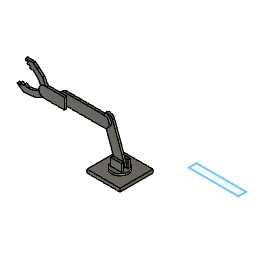
review_model_1 v2 (Autodesk Fusion 360 design; units mm, degrees)
Autodesk Fusion 360 part; units mm, degrees
note: some values were not read from the file. Set by a fixed rule: which sketch regions a step uses.
sketch "Sketch1" plane through (0, 0, 0) normal (0, 1, 0) x (1, 0, 0)
  line L0 (-108.5781, -41.3544) -> (68.499, -41.3544)
  line L1 (68.499, -41.3544) -> (68.499, 8.6456)
  line L2 (68.499, 8.6456) -> (-108.5781, 8.6456)
  line L3 (-108.5781, 8.6456) -> (-108.5781, -41.3544)
  circle A0 centre (-108.5781, -16.3544) radius 25
  circle A1 centre (68.499, -16.3544) radius 25
  circle A2 centre (-108.5781, -16.3544) radius 5
  circle A3 centre (68.499, -16.3544) radius 5
  dimension "d1" = 50
  dimension "d2" = 50
  dimension "d3" = 50
  dimension "d4" = 10
  dimension "d5" = 10
  constraint horizontal L0
  constraint vertical L1
  constraint horizontal L2
  constraint vertical L3
  constraint midpoint L3 A0.centre
  constraint midpoint L1 A1.centre
  constraint concentric A0 A2
  constraint concentric A1 A3
  measures "d1" distance of L0.start L2.end
  measures "d2" diameter of A0
  measures "d3" diameter of A1
  measures "d4" diameter of A2
  measures "d5" diameter of A3
extrude "Extrude1" add sketch "Sketch1" along normal blind 10 contours L0 L2 A0 A1 | L3 A0 A2 | L3 A0 A2 | L1 A1 A3 | L1 A1 A3 makes body 1
extrude "Extrude2" add sketch "Sketch1" along normal blind 10 and the other way blind 5 contours L3 A2 | L3 A2 bodies 1
extrude "Extrude3" add sketch "Sketch1" along normal blind 15 contours L1 A3 | L1 A3 bodies 1
sketch "Sketch2" plane through (0, 0, 0) normal (0, 0, 1) x (1, 0, 0)
  line L0 (-49.1019, 49.257) -> (100.8981, 49.257)
  line L1 (100.8981, 49.257) -> (100.8981, -100.743)
  line L2 (100.8981, -100.743) -> (-49.1019, -100.743)
  line L3 (-49.1019, -100.743) -> (-49.1019, 49.257)
  circle A0 centre (25.8981, -25.743) radius 37.5
  line L4 (44.4703, -49.3068) -> (33.9434, -49.3068)
  line L5 (33.9434, -49.3068) -> (33.9434, -0.5708)
  line L6 (33.9434, -0.5708) -> (44.4703, -0.5708)
  line L7 (44.4703, -0.5708) -> (44.4703, -49.3068)
  line L8 (14.9434, -49.3068) -> (4.8063, -49.3068)
  line L9 (4.8063, -49.3068) -> (4.8063, -0.5708)
  line L10 (4.8063, -0.5708) -> (14.9434, -0.5708)
  line L11 (14.9434, -0.5708) -> (14.9434, -49.3068)
  dimension "d14" = 150
  dimension "d15" = 150
  dimension "d19" = 75
  dimension "d24" = 19
  constraint horizontal L0
  constraint vertical L1
  constraint horizontal L2
  constraint vertical L3
  constraint horizontal L4
  constraint vertical L5
  constraint horizontal L6
  constraint vertical L7
  constraint horizontal L8
  constraint vertical L9
  constraint horizontal L10
  constraint vertical L11
  measures "d14" distance of L0.start L0.end
  measures "d15" distance of L0.start L2.end
  measures "d19" diameter of A0
  measures "d24" distance of L5 L11
copy_body "Body->Comp1" bodies 1 removing the originals makes body 2 in component "Component"
extrude "Extrude4" add sketch "Sketch2" along normal blind 15 separate body contours L0 L1 L2 L3 | A0 | L4 L5 L6 L7 | L8 L9 L10 L11 makes body 3
copy_body "Body->Comp2" bodies 3 removing the originals makes body 4 in component "Component'"
sketch "Sketch3" plane through (0, 0, 0) normal (0, 1, 0) x (1, 0, 0)
copy_body "CopyPasteBodies1" bodies 2 body 2 seen with x (1, 0, 0) y (0, 1, 0) z (0, 0, 1) at (-36.8422, -38.5395, 66.2192) makes body 5
move_body "Move1" bodies 5 to x (1, 0, 0) y (0, 1, 0) z (0, 0, 1) at (200.1869, 0, -32.8723)
copy_body "Body->Comp3" bodies 5 removing the originals makes body 6 in component "Component''"
move_body "Move1'" bodies 6 to x (0.34202, 0, -0.939693) y (0, 1, 0) z (0.939693, 0, 0.34202) at (73.7396, 0, 203.378) in component "Component''"
scale "Scale1" factor 0.881229 about (223.2311, -38.5395, 11.0656) bodies 6 in component "Component''"
extrude "Extrude1'" add sketch "Sketch2" along normal blind 10 and the other way blind -1 separate body contours A0 | L4 L5 L6 L7 | L8 L9 L10 L11 sketch seen with x (1, 0, 0) y (0, 1, 0) z (0, 0, 1) at (-0.0098, -0.0113, 15.0232) makes body 7 in component "Component'"
extrude "Extrude2'" add sketch "Sketch2" along normal blind 35 and the other way blind 5 contours L4 L5 L6 L7 | L8 L9 L10 L11 sketch seen with x (1, 0, 0) y (0, 1, 0) z (0, 0, 1) at (0.0483, -0.0113, 25.1603) bodies 7 in component "Component'"
copy_body "Body->Comp1'" bodies 7 removing the originals makes body 8 in component "Component'''"
sketch "Sketch4" plane through (0, 0, 0) normal (0, 1, 0) x (1, 0, 0)
  line L0 (94.4913, -79.8435) -> (4.0946, -79.8435)
  line L1 (4.0946, -79.8435) -> (4.0946, -29.8435)
  line L2 (4.0946, -29.8435) -> (94.4913, -29.8435)
  line L3 (94.4913, -29.8435) -> (94.4913, -79.8435)
  circle A0 centre (75.9076, -54.8435) radius 5
  circle A1 centre (4.0946, -54.8435) radius 25
  dimension "d29" = 50
  dimension "d30" = 10
  dimension "d55" = 50
  constraint horizontal L0
  constraint vertical L1
  constraint horizontal L2
  constraint vertical L3
  constraint midpoint L1 A1.centre
  measures "d29" distance of L0.start L2.end
  measures "d30" diameter of A0
  measures "d55" diameter of A1
extrude "Extrude5" add sketch "Sketch4" along normal blind 10 separate body makes body 9
extrude "Extrude6" add sketch "Sketch4" along normal blind 15 contours A0 bodies 9
copy_body "Body->Comp4" bodies 9 removing the originals makes body 10 in component "Component''''"
move_body "Move1''" bodies 8 to x (0, -1, 0) y (1, 0, 0) z (0, 0, 1) at (64.2053, 14.305, 0) in component "Component'''"
move_face "MoveFace1" to x (0.965926, 0, 0.258819) y (0, 1, 0) z (-0.258819, 0, 0.965926) at (14.8115, 0, 0.8453) 1 faces at (26.3656, 10, 54.8435) on bodies 10 in component "Component''''"
sketch "Sketch5" plane through (0, 0, 0) normal (0, 1, 0) x (1, 0, 0)
  line L0 (-153.4597, -52.3463) -> (-142.5808, -41.4675)
  line L1 (-142.5808, -41.4675) -> (-130.4737, -29.3604)
  line L2 (-130.4737, -29.3604) -> (-112.9272, -46.9069)
  line L3 (-112.9272, -46.9069) -> (-136.5273, -67.4364)
  line L4 (-112.9272, -46.9069) -> (-96.258, -16.5514)
  line L5 (-96.258, -16.5514) -> (-121.7004, -10.1329)
  line L6 (-121.7004, -10.1329) -> (-130.4737, -29.3604)
  circle A0 centre (-103.7737, 7.2921) radius 25
  line L7 (-153.4597, -52.3463) -> (-169.3332, -52.3463)
  line L8 (-169.3332, -52.3463) -> (-169.3332, -63.6855)
  line L9 (-169.3332, -63.6855) -> (-182.589, -63.6855)
  line L10 (-182.589, -63.6855) -> (-176.6061, -75.4928)
  line L11 (-176.6061, -75.4928) -> (-190.2211, -75.4928)
  line L12 (-190.2211, -75.4928) -> (-190.2211, -82.3641)
  line L13 (-190.2211, -82.3641) -> (-154.8723, -82.3641)
  line L14 (-154.8723, -82.3641) -> (-136.5273, -67.4364)
  point P0 (-121.7004, -10.1329)
  point P1 (-96.258, -16.5514)
  dimension "d56" = 50
  constraint perpendicular L1 L2
  constraint coincident P0 A0
  constraint coincident P0 L5.end
  constraint coincident P1 L4.end
  constraint coincident A0 P1
  constraint horizontal L7
  constraint perpendicular L7 L8
  constraint perpendicular L8 L9
  constraint perpendicular L8 L11
  constraint perpendicular L9 L12
  constraint perpendicular L12 L13
  measures "d56" diameter of A0
extrude "Extrude7" add sketch "Sketch5" along normal blind 10 separate body contours L0 L1 L2 L3 L7 L8 L9 L10 L11 L12 L13 L14 | L2 L4 L6 A0 makes body 11
copy_body "Body->Comp5" bodies 11 removing the originals makes body 12 in component "Component'''''"
copy_body "CopyPasteBodies2" bodies 12 makes body 13
move_body "Move2" bodies 13 to x (1, 0, 0) y (0, 1, 0) z (0, 0, 1) at (32.4935, 0, -22.4043)
copy_body "Body->Comp6" bodies 13 removing the originals makes body 14 in component "Component''''''"
move_body "Move1'''" bodies 12 to x (0.817287, 0.030154, -0.575442) y (0.122788, -0.984808, 0.122788) z (-0.562997, -0.17101, -0.808573) at (-25.596, 11.9543, -82.2192) in component "Component'''''"
sketch "Sketch6" plane through (0, 0, 0) normal (0, 0, 1) x (1, 0, 0)
  line L0 (186.303, 161.3111) -> (411.2298, 161.3111)
  line L1 (411.2298, 161.3111) -> (411.2298, 126.0953)
  line L2 (411.2298, 126.0953) -> (186.303, 126.0953)
  line L3 (186.303, 126.0953) -> (186.303, 161.3111)
  dimension "d69" = 224.9268
  constraint horizontal L0
  constraint vertical L1
  constraint horizontal L2
  constraint vertical L3
  measures "d69" distance of L0.start L0.end
component "Component" placed x (1, 0, 0) y (0, 1, 0) z (0, 0, 1) at (-95.2156, -47.4595, 146.6886)
component "Component'" placed x (1, 0, 0) y (0, 1, 0) z (0, 0, 1) at (-0.0483, 0.0113, -25.1603)
component "Component''" placed x (1, 0, 0) y (0, 1, 0) z (0, 0, 1) at (-175.8749, 10.4862, 12.8776)
component "Component''''" placed x (1, 0, 0) y (0, 1, 0) z (0, 0, 1) at (-279.7014, -67.4595, 108.1996)
component "Component'''''" placed x (0.992433, -0.122788, 0) y (0.121844, 0.984808, 0.123724) z (-0.015192, -0.122788, 0.992317) at (-171.5874, -84.0972, 178.2766)
component "Component''''''" placed x (1, 0, 0) y (0, 1, 0) z (0, 0, 1) at (-204.3267, -67.4595, 192.7394)
component "Component'''" placed x (1, 0, 0) y (0, 1, 0) z (0, 0, 1) at (-12.5529, -14.1595, -1.0232) in component "Component'"
